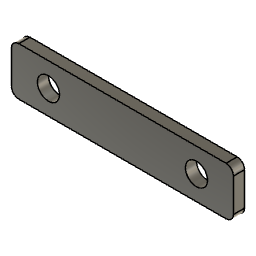
Pos11 (Autodesk Fusion 360 design; units mm, degrees)
Autodesk Fusion 360 part; units mm, degrees
sketch "Sketch1" plane through (0, 0, 0) normal (0, 1, 0) x (1, 0, 0)
  line L0 (28, 6.5) -> (-28, 6.5)
  line L1 (-30, 4.5) -> (-30, -4.5)
  line L2 (-28, -6.5) -> (28, -6.5)
  line L3 (30, -4.5) -> (30, 4.5)
  line L4 (30, 6.5) -> (-30, -6.5) construction
  line L5 (-30, 6.5) -> (30, -6.5) construction
  arc A0 (-30, -4.5) -> (-28, -6.5) centre (-28, -4.5) ccw
  arc A1 (28, -6.5) -> (30, -4.5) centre (28, -4.5) ccw
  arc A2 (30, 4.5) -> (28, 6.5) centre (28, 4.5) ccw
  arc A3 (-28, 6.5) -> (-30, 4.5) centre (-28, 4.5) ccw
  line L6 (0, 0) -> (20, 0) construction
  line L7 (0, 0) -> (-20, 0) construction
  circle A4 centre (20, 0) radius 3
  circle A5 centre (-20, 0) radius 3
  dimension "d1" = 60
  dimension "d2" = 13
  dimension "d3" = 2
  dimension "d4" = 2
  dimension "d5" = 20
  dimension "d6" = 20
  dimension "d7" = 6
  dimension "d8" = 6
  constraint horizontal L0
  constraint perpendicular L0 L1
  constraint parallel L0 L2
  constraint parallel L1 L3
  constraint coincident L4 L6.start
  constraint coincident L5 L6.start
  constraint coincident L6.start L7.start
  constraint coincident L4.end L2
  constraint coincident L4.end L1
  constraint tangent L2 A0
  constraint tangent L1 A0
  constraint coincident L5.end L2
  constraint coincident L5.end L3
  constraint tangent L2 A1
  constraint tangent L3 A1
  constraint coincident L4.start L3
  constraint coincident L4.start L0
  constraint tangent L3 A2
  constraint tangent L0 A2
  constraint equal A1 A2
  constraint coincident L5.start L0
  constraint coincident L5.start L1
  constraint tangent L0 A3
  constraint tangent L1 A3
  constraint equal A1 A3
  constraint horizontal L6
  constraint parallel L6 L7
  constraint coincident L6.end A4.centre
  constraint coincident L7.end A5.centre
  measures "d1" distance of L4.end L5.end
  measures "d2" distance of L4.start L5.end
  measures "d3" radius of A0
  measures "d4" radius of A1
  measures "d5" distance of L6.start L6.end
  measures "d6" distance of L6.start L7.end
  measures "d7" diameter of A4
  measures "d8" diameter of A5
extrude "Extrude1" add sketch "Sketch1" along normal blind 3
